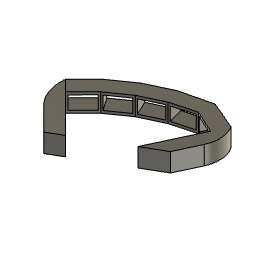
HandBaseP1 v4 (Autodesk Fusion 360 design; units mm, degrees)
Autodesk Fusion 360 part; units mm, degrees
sketch "Sketch1" plane through (0, 0, 0) normal (0, 0, 1) x (1, 0, 0)
  line L0 (0, 0) -> (5.6461, 5.6676)
  line L1 (5.6461, 5.6676) -> (12.1905, 10.2687)
  line L2 (12.1905, 10.2687) -> (19.4345, 13.6634)
  line L3 (19.4345, 13.6634) -> (27.158, 15.7487)
  line L4 (27.158, 15.7487) -> (34.4149, 12.3816)
  line L5 (0, 0) -> (-3.5423, 3.5288)
  line L6 (5.6461, 5.6676) -> (2.4248, 9.4917)
  line L7 (12.1905, 10.2687) -> (9.6823, 14.5941)
  line L8 (19.4345, 13.6634) -> (17.7155, 18.3586)
  line L9 (27.158, 15.7487) -> (27.5843, 20.7305)
  line L10 (34.4149, 12.3816) -> (36.5193, 16.9171)
  line L11 (-3.5423, 3.5288) -> (2.4248, 9.4917)
  line L12 (2.4248, 9.4917) -> (9.6823, 14.5941)
  line L13 (9.6823, 14.5941) -> (17.7155, 18.3586)
  line L14 (17.7155, 18.3586) -> (27.5843, 20.7305)
  line L15 (27.5843, 20.7305) -> (36.5193, 16.9171)
  line L16 (26.9936, -3.6128) -> (33.656, 0.2507)
  line L17 (12.1791, -12.2036) -> (7.7039, -14.7988)
  line L18 (7.7039, -14.7988) -> (0.3124, -7.4021)
  line L19 (-3.5423, 3.5288) -> (12.1791, -12.2036)
  line L20 (36.5193, 16.9171) -> (26.9936, -3.6128)
  line L21 (33.656, 0.2507) -> (37.0912, 7.6543)
  arc A0 (-3.5423, 3.5288) -> (0.3124, -7.4021) centre (9.8153, 2.0941) ccw
  arc A1 (37.0912, 7.6543) -> (36.5193, 16.9171) centre (28.2481, 11.7574) ccw
  line L22 (7.7039, -14.7988) -> (12.1791, -12.2036)
  line L23 (26.9936, -3.6128) -> (33.656, 0.2507)
  dimension "d1" = 170
  dimension "d2" = 170
  dimension "d3" = 170
  dimension "d4" = 140
  dimension "d5" = 8
  dimension "d6" = 8
  dimension "d7" = 8
  dimension "d8" = 8
  dimension "d9" = 8
  dimension "d10" = 5
  dimension "d11" = 5
  dimension "d12" = 5
  dimension "d13" = 5
  dimension "d14" = 5
  dimension "d15" = 5
  dimension "d16" = 95
  dimension "d17" = 95
  dimension "d18" = 95
  dimension "d19" = 110
  dimension "d24" = 30
  constraint coincident L0.start L5.start
  constraint perpendicular L0 L5
  constraint perpendicular L4 L10
  constraint perpendicular L11 L19
  constraint perpendicular L4 L20
  constraint parallel L16 L22
  constraint tangent L18 A0
  constraint tangent L21 A1
  constraint collinear L22 L23
  measures "d1" angle of L0 L1
  measures "d2" angle of L1 L2
  measures "d3" angle of L2 L3
  measures "d4" angle of L3 L4
  measures "d5" distance of L0.start L0.end
  measures "d6" distance of L1.end L2.end
  measures "d7" distance of L2.end L3.end
  measures "d8" distance of L3.end L4.end
  measures "d9" distance of L0.end L1.end
  measures "d10" distance of L0.start L5.end
  measures "d11" distance of L0.end L6.end
  measures "d12" distance of L1.end L7.end
  measures "d13" distance of L2.end L8.end
  measures "d14" distance of L3.end L9.end
  measures "d15" distance of L4.end L10.end
  measures "d16" angle of L0 L6
  measures "d17" angle of L1 L7
  measures "d18" angle of L2 L8
  measures "d19" angle of L3 L9
  measures "d24" distance of L17.end L16.end
extrude "Extrude1" add sketch "Sketch1" along normal blind 6
sketch "Sketch3" plane through (0, 0, 0) normal (0.708452, -0.705759, 0) x (0.705759, 0.708452, 0)
  line L0 (0, 0) -> (8, 0)
  line L1 (8, 0) -> (8, 6)
  line L2 (8, 6) -> (0, 6)
  line L3 (0, 6) -> (0, 0)
  line L4 (0.55, 5.15) -> (7.45, 5.15)
  line L5 (7.45, 5.15) -> (7.45, 0.85)
  line L6 (7.45, 0.85) -> (0.55, 0.85)
  line L7 (0.55, 0.85) -> (0.55, 5.15)
  dimension "d27" = 6.9
  dimension "d28" = 4.3
  dimension "d29" = 0.85
  dimension "d30" = 0.55
  constraint horizontal L4
  constraint vertical L5
  constraint horizontal L6
  constraint vertical L7
  measures "d27" distance of L5.end L6.end
  measures "d28" distance of L4.start L6.end
  measures "d29" distance of L0 L6
  measures "d30" distance of L3 L7
extrude "Extrude2" cut sketch "Sketch3" against normal blind 9 contours L4 L5 L6 L7
sketch "Sketch4" plane through (-0.799, 1.1364, 0) normal (0.575135, -0.818058, 0) x (0.818058, 0.575135, 0)
  line L0 (7.8785, 0) -> (15.8785, 0)
  line L1 (15.8785, 0) -> (15.8785, 6)
  line L2 (15.8785, 6) -> (7.8785, 6)
  line L3 (7.8785, 6) -> (7.8785, 0)
  line L4 (8.4285, 5.15) -> (15.3285, 5.15)
  line L5 (15.3285, 5.15) -> (15.3285, 0.85)
  line L6 (15.3285, 0.85) -> (8.4285, 0.85)
  line L7 (8.4285, 0.85) -> (8.4285, 5.15)
  dimension "d33" = 4.3
  dimension "d34" = 6.9
  dimension "d35" = 0.55
  dimension "d36" = 0.85
  constraint horizontal L4
  constraint vertical L5
  constraint horizontal L6
  constraint vertical L7
  measures "d33" distance of L4.start L6.end
  measures "d34" distance of L5.end L6.end
  measures "d35" distance of L3 L7
  measures "d36" distance of L0 L6
extrude "Extrude3" cut sketch "Sketch4" against normal blind 12 contours L4 L5 L6 L7
sketch "Sketch5" plane through (-1.7506, 3.7355, 0) normal (0.424343, -0.905501, 0) x (0.905501, 0.424343, 0)
  line L0 (15.396, 0) -> (23.396, 0)
  line L1 (23.396, 0) -> (23.396, 6)
  line L2 (23.396, 6) -> (15.396, 6)
  line L3 (15.396, 6) -> (15.396, 0)
  line L4 (15.946, 5.15) -> (22.846, 5.15)
  line L5 (22.846, 5.15) -> (22.846, 0.85)
  line L6 (22.846, 0.85) -> (15.946, 0.85)
  line L7 (15.946, 0.85) -> (15.946, 5.15)
  dimension "d39" = 6.9
  dimension "d40" = 4.3
  dimension "d41" = 0.55
  dimension "d42" = 0.85
  constraint horizontal L4
  constraint vertical L5
  constraint horizontal L6
  constraint vertical L7
  measures "d39" distance of L5.end L6.end
  measures "d40" distance of L4.start L6.end
  measures "d41" distance of L3 L7
  measures "d42" distance of L0 L6
extrude "Extrude4" cut sketch "Sketch5" against normal blind 10 contours L4 L5 L6 L7
sketch "Sketch6" plane through (-2.1179, 7.8445, 0) normal (0.260658, -0.965431, 0) x (0.965431, 0.260658, 0)
  line L0 (22.3242, 0) -> (30.3242, 0)
  line L1 (30.3242, 0) -> (30.3242, 6)
  line L2 (30.3242, 6) -> (22.3242, 6)
  line L3 (22.3242, 6) -> (22.3242, 0)
  line L4 (22.8742, 5.15) -> (29.7742, 5.15)
  line L5 (29.7742, 5.15) -> (29.7742, 0.85)
  line L6 (29.7742, 0.85) -> (22.8742, 0.85)
  line L7 (22.8742, 0.85) -> (22.8742, 5.15)
  dimension "d45" = 4.3
  dimension "d46" = 0.85
  dimension "d47" = 6.9
  dimension "d48" = 0.55
  constraint horizontal L4
  constraint vertical L5
  constraint horizontal L6
  constraint vertical L7
  measures "d45" distance of L4.start L6.end
  measures "d46" distance of L0 L6
  measures "d47" distance of L5.end L6.end
  measures "d48" distance of L3 L7
extrude "Extrude5" cut sketch "Sketch6" against normal blind 12 contours L4 L5 L6 L7
sketch "Sketch7" plane through (10.8238, 23.3276, 0) normal (-0.420892, -0.907111, 0) x (0.907111, -0.420892, 0)
  line L0 (18.0068, 0) -> (26.0068, 0)
  line L1 (26.0068, 0) -> (26.0068, 6)
  line L2 (26.0068, 6) -> (18.0068, 6)
  line L3 (18.0068, 6) -> (18.0068, 0)
  line L4 (18.5568, 5.15) -> (25.4568, 5.15)
  line L5 (25.4568, 5.15) -> (25.4568, 0.85)
  line L6 (25.4568, 0.85) -> (18.5568, 0.85)
  line L7 (18.5568, 0.85) -> (18.5568, 5.15)
  dimension "d51" = 4.3
  dimension "d52" = 6.9
  dimension "d53" = 0.55
  dimension "d54" = 0.85
  constraint horizontal L4
  constraint vertical L5
  constraint horizontal L6
  constraint vertical L7
  measures "d51" distance of L4.start L6.end
  measures "d52" distance of L5.end L6.end
  measures "d53" distance of L3 L7
  measures "d54" distance of L0 L6
extrude "Extrude6" cut sketch "Sketch7" against normal blind 15 contours L4 L5 L6 L7
